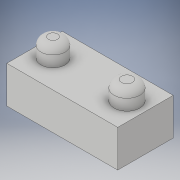
# Autodesk Inventor part: IR-Sensor
Saved by Autodesk Inventor 2019.5 (Build 235369000, 369)
## iProperties
Created: 2021-09-30
Part Number: IR-Sensor
Material: Generisch
Document SubType Name: Modeling
Designer: mritt
Density: 1 g/cm^3
Appearance: Vorgabe
Author: mritt
Autodesk Inventor part; units mm, degrees
ref_plane "YZ Plane" through (0, 0, 0) normal (1, 0, 0) x (0, 1, 0)
ref_plane "XZ Plane" through (0, 0, 0) normal (0, 1, 0) x (-1, 0, 0)
ref_plane "XY Plane" through (0, 0, 0) normal (0, 0, 1) x (1, 0, 0)
sketch "Skizze1" plane through (0, 0, 0) normal (0, 1, 0) x (-1, 0, 0)
  line L0 (22.6442, -7.5) -> (-7.3558, -7.5)
  line L1 (-7.3558, -7.5) -> (-7.3558, -22.5)
  line L2 (-7.3558, -22.5) -> (22.6442, -22.5)
  line L3 (22.6442, -22.5) -> (22.6442, -7.5)
  point P0 (0, 0)
  dimension "d0" = 15
  dimension "d1" = 30
  constraints: 8 end point, 2 parallel, 1 horizontal, 1 perpendicular
  measures "d0" distance of L2.end L0.start
  measures "d1" distance of L1.end L2.end
extrude "Extrusion1" add sketch "Skizze1" along normal blind 10
sketch "Skizze2" plane through (0, 10, 0) normal (0, 1, 0) x (1, 0, 0)
  circle A0 centre (-17.6442, 15) radius 3.2574
  circle A1 centre (2.3558, 15) radius 3.4818
  line L0 (-22.6442, 22.5) -> (-22.6442, 7.5) projected
  line L1 (7.3558, 7.5) -> (7.3558, 22.5) projected
  line L2 (7.3558, 22.5) -> (-22.6442, 22.5) projected
  point P0 (0, 0)
  dimension "d4" = 5
  dimension "d5" = 5
  dimension "d6" = 7.5
  dimension "d7" = 7.5
  constraints: 2 centre point
  measures "d4" distance from line of A0.centre L0
  measures "d5" distance from line of A1.centre L1
  measures "d6" distance from line of A1.centre L2
  measures "d7" distance from line of A0.centre L2
extrude "Extrusion2" add sketch "Skizze2" along normal blind 5
fillet "Rundung1" radius 2 2 edges at (-20.9017, 15, -15) (-1.1261, 15, -15)
